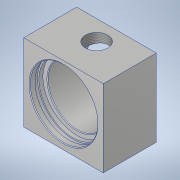
# Autodesk Inventor part: Sensoraufnahme
Saved by Autodesk Inventor 2021 (Build 250183000, 183)
## iProperties
Created: 2021-04-27
Part Number: Sensoraufnahme
Material: Aluminium 6061
Document SubType Name: Modeling
Designer: Michael
Density: 2.7 g/cm^3
Appearance: Aluminium - flach
Author: Michael
Autodesk Inventor part; units mm, degrees
ref_plane "YZ Plane" through (0, 0, 0) normal (1, 0, 0) x (0, 1, 0)
ref_plane "XZ Plane" through (0, 0, 0) normal (0, 1, 0) x (-1, 0, 0)
ref_plane "XY Plane" through (0, 0, 0) normal (0, 0, 1) x (1, 0, 0)
sketch "Skizze5" plane through (0, 0, 0) normal (0, 0, 1) x (1, 0, 0)
  circle A0 centre (0, 0) radius 22
  line L0 (-30, 28.25) -> (30, 28.25)
  line L1 (30, 28.25) -> (30, -28.25)
  line L2 (30, -28.25) -> (-30, -28.25)
  line L3 (-30, -28.25) -> (-30, 28.25)
  dimension "d26" = 44
  dimension "d27" = 60
  dimension "d28" = 56.5
  dimension "d29" = 30
  dimension "d30" = 28.25
  constraints: 8 end point, 2 parallel, 1 centre point, 1 coincident, 1 horizontal, 1 perpendicular
  measures "d26" diameter of A0
  measures "d27" distance of L0.start L0.end
  measures "d28" distance of L0.end L1.end
  measures "d29" distance from line of L1 point (0, 0)
  measures "d30" distance from line of L2 point (0, 0)
extrude "Extrusion2" add sketch "Skizze5" along normal blind 40
sketch "Skizze6" plane through (-30, 28.25, 0) normal (0, 1, 0) x (1, 0, 0)
  line L0 (60, -40) -> (0, -40) projected
  line L1 (60, 0) -> (60, -40) projected
  point P0 (30, 0)
  point P1 (30, -15)
  dimension "d34" = 30
  dimension "d73" = 15
  measures "d34" distance from line of L1 point (30, -15)
  measures "d73" distance of point (30, -15) point (30, 0)
hole "Bohrung3" at (0, 28.25, 15) direction (0, -1, 0) diameter 16.918 depth 41.1 tip angle 118 thread size "M18x1" class "6H" standard "ISO Metric profile"
sketch "Skizze7" plane through (0, 0, 40) normal (0, 0, 1) x (1, 0, 0)
  circle A0 centre (0, 0) radius 25.5
  dimension "d42" = 51
  constraints: 1 centre point, 1 coincident
  measures "d42" diameter of A0
extrude "Extrusion3" cut sketch "Skizze7" against normal blind 10
chamfer "Fase1" distance 0.5 angle 45 3 edges at (-25.5, 0, 40) (-22, 0, 30) (-22, 0, 0)
sketch "Skizze9" plane through (0, 0, 0) normal (0, 0, -1) x (-1, 0, 0)
  line L0 (30, 28.25) -> (-30, 28.25) projected
  line L1 (30, -28.25) -> (30, 28.25) projected
  point P0 (0, 0)
  point P1 (-24, -24)
  point P2 (-24, 22.25)
  point P3 (24, 22.25)
  point P4 (24, -24)
  dimension "d77" = 46.25
  dimension "d78" = 48
  dimension "d79" = 6
  dimension "d80" = 6
  constraints: 2 horizontal alignment, 2 vertical alignment
  measures "d77" distance of point (24, 22.25) point (24, -24)
  measures "d78" distance of point (-24, 22.25) point (24, 22.25)
  measures "d79" distance from line of L0 point (24, 22.25)
  measures "d80" distance from line of point (24, 22.25) L1
hole "Bohrung6" at (24, -24, 0) at (24, 22.25, 0) at (-24, 22.25, 0) at (-24, -24, 0) direction (0, 0, 1) diameter 4.134 depth 14.2 tip angle 118 thread size "M5x0.8" class "6H" standard "ISO Metric profile"
sketch "Skizze10" plane through (-30, -28.25, 0) normal (0, -1, 0) x (1, 0, 0)
  line L0 (60, 0) -> (0, 0) projected
  line L1 (0, 40) -> (60, 40) projected
  line L2 (0, 0) -> (60, 0)
  line L3 (60, 0) -> (60, 40)
  line L4 (60, 40) -> (0, 40)
  line L5 (0, 40) -> (0, 0)
  point P0 (30, 0)
  constraints: 8 end point, 2 parallel, 1 horizontal, 1 perpendicular
extrude "Extrusion4" add sketch "Skizze10" along normal blind 1.75
sketch "Skizze11" plane through (0, 0, 0) normal (0, 1, 0) x (-1, 0, 0)
  line L0 (-26.5, 36) -> (-25, 36)
  line L1 (-25, 36) -> (-25, 33)
  line L2 (-25, 33) -> (-26.5, 33)
  line L3 (-26.5, 33) -> (-26.5, 36)
  line L4 (0, -8) -> (0, 48) projected
  point P0 (0, 0)
  dimension "d90" = 1.5
  dimension "d91" = 25
  dimension "d92" = 33
  dimension "d93" = 3
  constraints: 8 end point, 2 parallel, 1 horizontal, 1 perpendicular
  measures "d90" distance of L1.end L2.end
  measures "d91" distance from line of L1 point (0, 0)
  measures "d92" distance from line of L2 point (0, 0)
  measures "d93" distance of L0.end L1.end
revolve "Umdrehung1" cut sketch "Skizze11" angle 360 about axis through (0, 0, -10) along (0, 0, 1)
equation "\"d29\" = 0.5 * d27"
equation "\"d30\" = 0.5 * d28"
